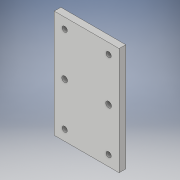
# Autodesk Inventor part: yCarraige
Saved by Autodesk Inventor 2019 (Build 230136000, 136)
## iProperties
Created: 2019-05-08
Part Number: yCarraige
Material: Generic
Document SubType Name: Modeling
Designer: Alex Jones
Density: 1 g/cm^3
Appearance: Default
Author: Alex Jones
Autodesk Inventor part; units mm, degrees
ref_plane "YZ Plane" through (0, 0, 0) normal (1, 0, 0) x (0, 1, 0)
ref_plane "XZ Plane" through (0, 0, 0) normal (0, 1, 0) x (-1, 0, 0)
ref_plane "XY Plane" through (0, 0, 0) normal (0, 0, 1) x (1, 0, 0)
sketch "Sketch1" plane through (0, 0, 0) normal (0, 0, 1) x (1, 0, 0)
  circle A0 centre (-610.4613, 17.8) radius 2.5 projected
  circle A1 centre (-610.4613, 17.8) radius 9.9 construction
  circle A2 centre (-652.4613, 17.8) radius 2.5 projected
  circle A3 centre (-652.4613, 17.8) radius 9.9 construction
  circle A4 centre (-610.4613, -65) radius 2.5 projected
  circle A5 centre (-610.4613, -65) radius 9.9 construction
  circle A6 centre (-652.4613, -65) radius 2.5 projected
  circle A7 centre (-652.4613, -65) radius 9.9 construction
  line L0 (-610.4613, -65) -> (-652.4613, -65) construction
  line L1 (-652.4613, -65) -> (-652.4613, 17.8) construction
  line L2 (-652.4613, 17.8) -> (-610.4613, 17.8) construction
  line L3 (-610.4613, 17.8) -> (-610.4613, -65) construction
  line L4 (-662.4613, -75) -> (-600.4613, -75)
  line L5 (-600.4613, -75) -> (-600.4613, 27.8)
  line L6 (-600.4613, 27.8) -> (-662.4613, 27.8)
  line L7 (-662.4613, 27.8) -> (-662.4613, -75)
  point P0 (0, 0)
  dimension "d0" = 10
  constraints: 16 end point, 4 parallel, 2 perpendicular, 1 horizontal, 3 other
  measures "d0" distance between parallel lines of L0 L4
extrude "Extrusion1" add sketch "Sketch1" along normal blind 6.35
sketch "Sketch2" plane through (0, 0, 6.35) normal (0, 0, 1) x (1, 0, 0)
  circle A0 centre (-610.4613, 17.8) radius 2.5 projected
  circle A1 centre (-610.4613, -65) radius 2.5 projected
  circle A2 centre (-652.4613, -65) radius 2.5 projected
  circle A3 centre (-652.4613, 17.8) radius 2.5 projected
  circle A4 centre (-652.4613, 17.8) radius 2.5 projected
  line L0 (-652.4613, 17.8) -> (-652.4613, -65) construction
  circle A5 centre (-610.4613, 17.8) radius 2.5 projected
  circle A6 centre (-610.4613, -65) radius 2.5 projected
  line L1 (-610.4613, 17.8) -> (-610.4613, -65) construction
  circle A7 centre (-610.4613, -23.6) radius 2.75
  circle A8 centre (-652.4613, -23.6) radius 2.75
  point P0 (0, 0)
  dimension "d3" = 5.5
  constraints: 4 end point, 2 centre point, 2 midpoint, 2 vertical, 1 equal radius
  measures "d3" diameter of A8
extrude "Extrusion2" cut sketch "Sketch2" against normal blind 25.4 contours A7 | A8
body "Solid1"
